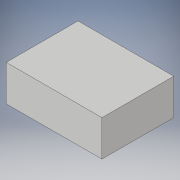
# Autodesk Inventor part: BS #1
Saved by Autodesk Inventor 2019 (Build 230136000, 136)
## iProperties
Created: 2019-02-18
Part Number: BS #1
Material: Generic
Document SubType Name: Modeling
Designer: Tesler
Density: 1 g/cm^3
Appearance: Default
Author: Tesler
Autodesk Inventor part; units mm, degrees
ref_plane "YZ Plane" through (0, 0, 0) normal (1, 0, 0) x (0, 1, 0)
ref_plane "XZ Plane" through (0, 0, 0) normal (0, 1, 0) x (-1, 0, 0)
ref_plane "XY Plane" through (0, 0, 0) normal (0, 0, 1) x (1, 0, 0)
sketch "Sketch1" plane through (0, 0, 0) normal (0, 1, 0) x (-1, 0, 0)
  line L0 (0, 0) -> (203.2, 0)
  line L1 (203.2, 0) -> (203.2, -152.4)
  line L2 (203.2, -152.4) -> (0, -152.4)
  line L3 (0, -152.4) -> (0, 0)
  dimension "d0" = 203.2
  dimension "d1" = 152.4
  constraints: 8 end point, 2 parallel, 1 horizontal, 1 perpendicular
  measures "d0" distance of L1.end L2.end
  measures "d1" distance of L0.end L1.end
extrude "Extrusion1" add sketch "Sketch1" along normal blind 76.2
sketch "Sketch2" plane through (0, 0, 0) normal (0, -1, 0) x (1, 0, 0)
  line L0 (-190.5, -6.35) -> (-12.7, -6.35)
  line L1 (-12.7, -6.35) -> (-12.7, -19.05)
  line L2 (-12.7, -19.05) -> (-190.5, -19.05)
  line L3 (-190.5, -19.05) -> (-190.5, -6.35)
  line L4 (-190.5, -133.35) -> (-12.7, -133.35)
  line L5 (-12.7, -133.35) -> (-12.7, -146.05)
  line L6 (-12.7, -146.05) -> (-190.5, -146.05)
  line L7 (-190.5, -146.05) -> (-190.5, -133.35)
  line L8 (0, -152.4) -> (0, 0) projected
  line L9 (-203.2, 0) -> (-203.2, -152.4) projected
  line L10 (-203.2, -152.4) -> (0, -152.4) projected
  line L11 (0, 0) -> (-203.2, 0) projected
  dimension "d4" = 12.7
  dimension "d5" = 12.7
  dimension "d6" = 12.7
  dimension "d7" = 12.7
  dimension "d8" = 6.35
  dimension "d9" = 6.35
  dimension "d10" = 12.7
  dimension "d11" = 12.7
  constraints: 16 end point, 4 parallel, 2 horizontal, 2 perpendicular
  measures "d4" distance between parallel lines of L8 L5
  measures "d5" distance between parallel lines of L9 L7
  measures "d6" distance between parallel lines of L9 L3
  measures "d7" distance between parallel lines of L8 L1
  measures "d8" distance between parallel lines of L10 L6
  measures "d9" distance between parallel lines of L11 L0
  measures "d10" distance between parallel lines of L6 L4
  measures "d11" distance between parallel lines of L0 L2
extrude "Extrusion2" cut sketch "Sketch2" against normal blind 6.35 contours L0 L1 L2 L3 | L4 L5 L6 L7
body "Solid1"
